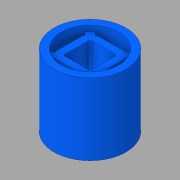
# Autodesk Inventor part: gear_collar_small
Saved by Autodesk Inventor 2019.3 (Build 233278000, 278)
## iProperties
Created: 2019-01-25
Part Number: gear_collar_small
Material: Generic
Document SubType Name: Modeling
Designer: Varga Daniel
Density: 1 g/cm^3
Appearance: Blue - 285 C
Author: Varga Daniel
Autodesk Inventor part; units mm, degrees
ref_plane "YZ Plane" through (0, 0, 0) normal (1, 0, 0) x (0, 1, 0)
ref_plane "XZ Plane" through (0, 0, 0) normal (0, 1, 0) x (-1, 0, 0)
ref_plane "XY Plane" through (0, 0, 0) normal (0, 0, 1) x (1, 0, 0)
derived "Base_part.ipt"
sketch "Axle_hole_sketch" plane through (0, 0, 0) normal (0, 1, 0) x (-1, 0, 0)
  line L0 (-14.3207, 2.4447) -> (-17.4707, 2.4447)
  line L1 (-17.7707, 2.7447) -> (-17.7707, 5.8947)
  line L2 (-17.4707, 6.1947) -> (-14.3207, 6.1947)
  line L3 (-14.0207, 5.8947) -> (-14.0207, 2.7447)
  line L4 (-14.0207, 2.4447) -> (-17.7707, 6.1947) construction
  line L5 (-17.7707, 2.4447) -> (-14.0207, 6.1947) construction
  arc A0 (-14.3207, 2.4447) -> (-14.0207, 2.7447) centre (-14.3207, 2.7447) ccw
  arc A1 (-17.7707, 2.7447) -> (-17.4707, 2.4447) centre (-17.4707, 2.7447) ccw
  arc A2 (-17.4707, 6.1947) -> (-17.7707, 5.8947) centre (-17.4707, 5.8947) ccw
  arc A3 (-14.0207, 5.8947) -> (-14.3207, 6.1947) centre (-14.3207, 5.8947) ccw
  point P0 (0, 0)
  point P1 (-15.8957, 4.3197)
  dimension "d17" = 3.75
  dimension "d18" = 0.3
  dimension "d19" = 3.75
  measures "d17" distance between parallel lines of L3 L1
  measures "d18" radius of A3
  measures "d19" distance between parallel lines of L0 L2
sketch "Sketch1" plane through (0, 0, 0) normal (0, 1, 0) x (-1, 0, 0)
  circle A0 centre (0, 0) radius 6.5
  dimension "d2" = 13
  constraints: 1 centre point, 1 coincident
  measures "d2" diameter of A0
extrude "Extrusion1" [suppressed]
sketch "Sketch2" plane through (0, 2.5, 0) normal (0, 1, 0) x (1, 0, 0)
  line L0 (-1.575, -1.875) -> (1.575, -1.875)
  line L1 (1.875, -1.575) -> (1.875, 1.575)
  line L2 (1.575, 1.875) -> (-1.575, 1.875)
  line L3 (-1.875, 1.575) -> (-1.875, -1.575)
  line L4 (-1.875, -1.875) -> (1.875, 1.875) construction
  line L5 (1.875, -1.875) -> (-1.875, 1.875) construction
  arc A0 (-1.575, 1.875) -> (-1.875, 1.575) centre (-1.575, 1.575) ccw
  arc A1 (-1.875, -1.575) -> (-1.575, -1.875) centre (-1.575, -1.575) ccw
  arc A2 (1.575, -1.875) -> (1.875, -1.575) centre (1.575, -1.575) ccw
  arc A3 (1.875, 1.575) -> (1.575, 1.875) centre (1.575, 1.575) ccw
  line L6 (14.3207, -2.4447) -> (17.4707, -2.4447) construction
  line L7 (14.0207, -5.8947) -> (14.0207, -2.7447) construction
  arc A4 (14.3207, -2.4447) -> (14.0207, -2.7447) centre (14.3207, -2.7447) ccw construction
  line L8 (17.7707, -2.7447) -> (17.7707, -5.8947) construction
  arc A5 (17.7707, -2.7447) -> (17.4707, -2.4447) centre (17.4707, -2.7447) ccw construction
  arc A6 (17.4707, -6.1947) -> (17.7707, -5.8947) centre (17.4707, -5.8947) ccw construction
  line L9 (17.4707, -6.1947) -> (14.3207, -6.1947) construction
  arc A7 (14.0207, -5.8947) -> (14.3207, -6.1947) centre (14.3207, -5.8947) ccw construction
  point P0 (0, 0)
  dimension "d5" = 3.75
  dimension "d6" = 3.75
  dimension "d7" = 0.3
  dimension "d15" = 3.75
  dimension "d16" = 0.3
  constraints: 12 end point, 8 point on circle, 8 point on line, 8 tangent, 4 centre point, 3 equal radius, 2 midpoint, 2 parallel, 1 horizontal, 1 perpendicular
  measures "d5" distance of L5.end L4.end
  measures "d6" distance between parallel lines of L0 L2
  measures "d7" radius of A0
  measures "d15" distance between parallel lines of L7 L8
  measures "d16" radius of A5
extrude "Extrusion2" [suppressed]
sketch "Sketch3" plane through (0, 2.5, 0) normal (0, 1, 0) x (1, 0, 0)
  circle A0 centre (0, 0) radius 4
  dimension "d10" = 8
  constraints: 1 centre point, 1 coincident
  measures "d10" diameter of A0
extrude "Extrusion3" [suppressed]
fillet "Fillet1" [suppressed]
sketch "Sketch5" plane through (0, 0, 0) normal (0, 1, 0) x (-1, 0, 0)
  line L0 (1.575, 1.875) -> (-1.575, 1.875)
  line L1 (-1.875, 1.575) -> (-1.875, -1.575)
  line L2 (-1.575, -1.875) -> (1.575, -1.875)
  line L3 (1.875, -1.575) -> (1.875, 1.575)
  line L4 (1.875, 1.875) -> (-1.875, -1.875) construction
  line L5 (-1.875, 1.875) -> (1.875, -1.875) construction
  arc A0 (1.875, 1.575) -> (1.575, 1.875) centre (1.575, 1.575) ccw
  arc A1 (1.575, -1.875) -> (1.875, -1.575) centre (1.575, -1.575) ccw
  arc A2 (-1.875, -1.575) -> (-1.575, -1.875) centre (-1.575, -1.575) ccw
  arc A3 (-1.575, 1.875) -> (-1.875, 1.575) centre (-1.575, 1.575) ccw
  circle A4 centre (0, 0) radius 4
  circle A5 centre (0, 0) radius 5
  line L6 (1.575, -2.875) -> (-1.575, -2.875)
  arc A6 (-2.875, -1.575) -> (-1.575, -2.875) centre (-1.575, -1.575) ccw
  line L7 (-2.875, -1.575) -> (-2.875, 1.575)
  arc A7 (-1.575, 2.875) -> (-2.875, 1.575) centre (-1.575, 1.575) ccw
  line L8 (-1.575, 2.875) -> (1.575, 2.875)
  arc A8 (2.875, 1.575) -> (1.575, 2.875) centre (1.575, 1.575) ccw
  line L9 (2.875, 1.575) -> (2.875, -1.575)
  arc A9 (1.575, -2.875) -> (2.875, -1.575) centre (1.575, -1.575) ccw
  line L10 (-2.7771, -2.07) -> (-3.1598, -2.4527)
  line L11 (-2.07, -2.7771) -> (-2.4527, -3.1598)
  line L12 (3.1598, 2.4527) -> (2.7771, 2.07)
  line L13 (2.4527, 3.1598) -> (2.07, 2.7771)
  line L14 (3.1598, -2.4527) -> (2.7771, -2.07)
  line L15 (2.07, -2.7771) -> (2.4527, -3.1598)
  line L16 (-2.07, 2.7771) -> (-2.4527, 3.1598)
  line L17 (-2.7771, 2.07) -> (-3.1598, 2.4527)
  dimension "d20" = 3.75
  dimension "d21" = 3.75
  dimension "d22" = 0.3
  dimension "d23" = 1
  dimension "d24" = 1
  dimension "d25" = 10
  dimension "d26" = 1
  dimension "d27" = 1
  constraints: 36 end point, 24 point on circle, 9 centre point, 8 parallel, 8 point on line, 8 tangent, 4 collinear, 3 equal radius, 2 coincident, 2 midpoint, 2 perpendicular, 1 horizontal, 19 other
  measures "d20" distance between parallel lines of L3 L1
  measures "d21" distance between parallel lines of L2 L0
  measures "d22" radius of A0
  measures "d23" distance between parallel lines of L2 L6
  measures "d25" diameter of A5
  measures "d26" distance between parallel lines of L10 L11
  measures "d27" distance between parallel lines of L15 L14
extrude "Extrusion4" add sketch "Sketch5" along normal mid plane 8.4 contours L12 A8 L13 A4 | A4 L15 A9 L14 | A8 L9 A9 L6 A6 L7 A7 L8 | L16 A7 L17 A4 | A4 L10 A6 L11
extrude "Extrusion5" add sketch "Sketch5" along normal blind 1 contours A4 L14 A9 L9 A8 L12 | L13 A8 L8 A7 L16 A4 | A4 L11 A6 L6 A9 L15 | L17 A7 L7 A6 L10 A4
extrude "Extrusion6" add sketch "Sketch5" along normal mid plane 10 contours A5
equation "\"d5\" = d15"
equation "\"d6\" = d5"
equation "\"d7\" = d16"
equation "\"d20\" = d17"
equation "\"d21\" = d19"
equation "\"d22\" = d18"
equation "\"d23\" = Inner_route_thickness"
equation "\"d24\" = Wall_thickness"
equation "\"d26\" = Inner_route_thickness"
equation "\"d27\" = Inner_route_thickness"
equation "\"d28\" = Hole_height"
equation "\"d30\" = Inner_thickness"
equation "\"d32\" = Overall_height"
equation "\"Inner_route_thickness\" = 1"
equation "\"Wall_thickness\" = 1"
equation "\"Hole_height\" = 8.4"
equation "\"Inner_thickness\" = 1"
equation "\"Overall_height\" = 10"
body "Solid1"
